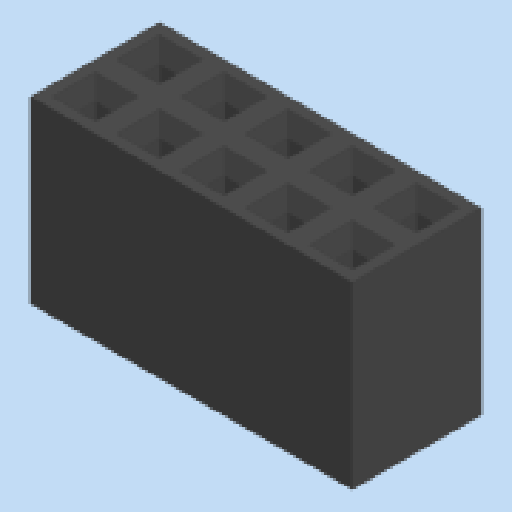
# Autodesk Inventor part: 2x5_P2.54mm_female_header
Saved by Autodesk Inventor 2024 (Build 280153000, 153)
## iProperties
Created: 2025-05-08
Part Number: 2x5_P2.54mm_female_header
Material: Generic
Document SubType Name: Modeling
Designer: XxPan
Density: 1 g/cm^3
Appearance: Default
Author: XxPan
Autodesk Inventor part; units mm, degrees
ref_plane "YZ Plane" through (0, 0, 0) normal (1, 0, 0) x (0, 1, 0)
ref_plane "XZ Plane" through (0, 0, 0) normal (0, 1, 0) x (-1, 0, 0)
ref_plane "XY Plane" through (0, 0, 0) normal (0, 0, 1) x (1, 0, 0)
sketch "Sketch1" plane through (0, 0, 0) normal (0, 1, 0) x (-1, 0, 0)
  line L0 (0, 0) -> (12.7, 0)
  line L1 (12.7, 0) -> (12.7, -5.08)
  line L2 (12.7, -5.08) -> (0, -5.08)
  line L3 (0, -5.08) -> (0, 0)
  line L4 (11.08, -0.92) -> (11.78, -0.92)
  line L5 (11.78, -0.92) -> (11.78, -1.62)
  line L6 (11.78, -1.62) -> (11.08, -1.62)
  line L7 (11.08, -1.62) -> (11.08, -0.92)
  line L8 (11.08, -0.92) -> (11.78, -1.62) construction
  line L9 (11.78, -0.92) -> (11.08, -1.62) construction
  line L10 (11.08, -3.46) -> (11.78, -3.46)
  line L11 (11.78, -3.46) -> (11.78, -4.16)
  line L12 (11.78, -4.16) -> (11.08, -4.16)
  line L13 (11.08, -4.16) -> (11.08, -3.46)
  line L14 (11.08, -3.46) -> (11.78, -4.16) construction
  line L15 (11.78, -3.46) -> (11.08, -4.16) construction
  line L16 (8.54, -0.92) -> (9.24, -0.92)
  line L17 (9.24, -0.92) -> (9.24, -1.62)
  line L18 (9.24, -1.62) -> (8.54, -1.62)
  line L19 (8.54, -1.62) -> (8.54, -0.92)
  line L20 (8.54, -0.92) -> (9.24, -1.62) construction
  line L21 (9.24, -0.92) -> (8.54, -1.62) construction
  line L22 (8.54, -3.46) -> (9.24, -3.46)
  line L23 (9.24, -3.46) -> (9.24, -4.16)
  line L24 (9.24, -4.16) -> (8.54, -4.16)
  line L25 (8.54, -4.16) -> (8.54, -3.46)
  line L26 (8.54, -3.46) -> (9.24, -4.16) construction
  line L27 (9.24, -3.46) -> (8.54, -4.16) construction
  line L28 (6, -0.92) -> (6.7, -0.92)
  line L29 (6.7, -0.92) -> (6.7, -1.62)
  line L30 (6.7, -1.62) -> (6, -1.62)
  line L31 (6, -1.62) -> (6, -0.92)
  line L32 (6, -0.92) -> (6.7, -1.62) construction
  line L33 (6.7, -0.92) -> (6, -1.62) construction
  line L34 (6, -3.46) -> (6.7, -3.46)
  line L35 (6.7, -3.46) -> (6.7, -4.16)
  line L36 (6.7, -4.16) -> (6, -4.16)
  line L37 (6, -4.16) -> (6, -3.46)
  line L38 (6, -3.46) -> (6.7, -4.16) construction
  line L39 (6.7, -3.46) -> (6, -4.16) construction
  line L40 (3.46, -0.92) -> (4.16, -0.92)
  line L41 (4.16, -0.92) -> (4.16, -1.62)
  line L42 (4.16, -1.62) -> (3.46, -1.62)
  line L43 (3.46, -1.62) -> (3.46, -0.92)
  line L44 (3.46, -0.92) -> (4.16, -1.62) construction
  line L45 (4.16, -0.92) -> (3.46, -1.62) construction
  line L46 (3.46, -3.46) -> (4.16, -3.46)
  line L47 (4.16, -3.46) -> (4.16, -4.16)
  line L48 (4.16, -4.16) -> (3.46, -4.16)
  line L49 (3.46, -4.16) -> (3.46, -3.46)
  line L50 (3.46, -3.46) -> (4.16, -4.16) construction
  line L51 (4.16, -3.46) -> (3.46, -4.16) construction
  line L52 (0.92, -0.92) -> (1.62, -0.92)
  line L53 (1.62, -0.92) -> (1.62, -1.62)
  line L54 (1.62, -1.62) -> (0.92, -1.62)
  line L55 (0.92, -1.62) -> (0.92, -0.92)
  line L56 (0.92, -0.92) -> (1.62, -1.62) construction
  line L57 (1.62, -0.92) -> (0.92, -1.62) construction
  line L58 (0.92, -3.46) -> (1.62, -3.46)
  line L59 (1.62, -3.46) -> (1.62, -4.16)
  line L60 (1.62, -4.16) -> (0.92, -4.16)
  line L61 (0.92, -4.16) -> (0.92, -3.46)
  line L62 (0.92, -3.46) -> (1.62, -4.16) construction
  line L63 (1.62, -3.46) -> (0.92, -4.16) construction
  point P0 (11.43, -1.27)
  point P1 (11.43, -3.81)
  point P2 (8.89, -1.27)
  point P3 (8.89, -3.81)
  point P4 (6.35, -1.27)
  point P5 (6.35, -3.81)
  point P6 (3.81, -1.27)
  point P7 (3.81, -3.81)
  point P8 (1.27, -1.27)
  point P9 (1.27, -3.81)
  dimension "d0" = 12.7
  dimension "d1" = 5.08
  dimension "d2" = 0.7
  dimension "d3" = 0.7
  dimension "d6" = 2.54
  dimension "d9" = 2.54
  dimension "d12" = 1.27
  dimension "d13" = 1.27
  constraints: 128 end point, 4 parallel, 3 horizontal, 2 collinear, 2 midpoint, 2 perpendicular, 1 vertical, 97 other
  measures "d0" distance of L1.end L2.end
  measures "d1" distance of L0.end L1.end
  measures "d2" distance of L5.end L6.end
  measures "d3" distance of L4.end L5.end
  measures "d6" distance of L4.start L10.start
  measures "d9" distance of L4.start L16.start
  measures "d12" distance from line of L1 point (11.43, -1.27)
  measures "d13" distance from line of L0 point (11.43, -1.27)
extrude "Extrusion1" add sketch "Sketch1" along normal blind 7.1
chamfer "Chamfer1" distance 0.5 angle 45 40 edges at (-8.89, 7.1, -4.16) (-9.24, 7.1, -3.81) (-8.89, 7.1, -3.46) (-8.54, 7.1, -3.81) (-11.08, 7.1, -3.81) (-11.43, 7.1, -3.46) (-11.78, 7.1, -3.81) (-11.43, 7.1, -4.16) (-11.08, 7.1, -1.27) (-11.43, 7.1, -1.62) (-11.78, 7.1, -1.27) (-11.43, 7.1, -0.92) (-9.24, 7.1, -1.27) (-8.89, 7.1, -0.92) (-8.89, 7.1, -1.62) (-8.54, 7.1, -1.27) (-6.7, 7.1, -1.27) (-6.35, 7.1, -0.92) (-6.35, 7.1, -1.62) (-6, 7.1, -1.27) (-6.35, 7.1, -3.46) (-6.7, 7.1, -3.81) (-6.35, 7.1, -4.16) (-6, 7.1, -3.81) (-3.81, 7.1, -4.16) (-4.16, 7.1, -3.81) (-3.81, 7.1, -3.46) (-3.46, 7.1, -3.81) (-4.16, 7.1, -1.27) (-3.81, 7.1, -1.62) (-3.46, 7.1, -1.27) (-3.81, 7.1, -0.92) (-1.62, 7.1, -1.27) (-1.27, 7.1, -1.62) (-0.92, 7.1, -1.27) (-1.27, 7.1, -0.92) (-1.27, 7.1, -3.46) (-1.62, 7.1, -3.81) (-1.27, 7.1, -4.16) (-0.92, 7.1, -3.81)
equation "\"d2\" = d3"
equation "\"d12\" = d13"
body "Solid1"
